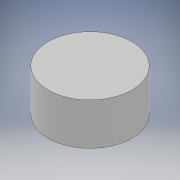
# Autodesk Inventor part: WesRoboticsInvention2019
Saved by Autodesk Inventor 2017 (Build 210142000, 142)
## iProperties
Created: 2019-11-21
Part Number: WesRoboticsInvention2019
Material: Generic
Document SubType Name: Modeling
Designer: Wes
Density: 1 g/cm^3
Appearance: Default
Author: Wes
Autodesk Inventor part; units mm, degrees
ref_plane "YZ Plane" through (0, 0, 0) normal (1, 0, 0) x (0, 1, 0)
ref_plane "XZ Plane" through (0, 0, 0) normal (0, 1, 0) x (-1, 0, 0)
ref_plane "XY Plane" through (0, 0, 0) normal (0, 0, 1) x (1, 0, 0)
sketch "Sketch1" plane through (0, 0, 0) normal (0, 0, 1) x (1, 0, 0)
  circle A0 centre (0, 0) radius 10
  dimension "d0" = 20
  constraints: 1 centre point, 1 coincident
  measures "d0" diameter of A0
extrude "Extrusion1" add sketch "Sketch1" along normal mid plane 10
body "Solid1"
